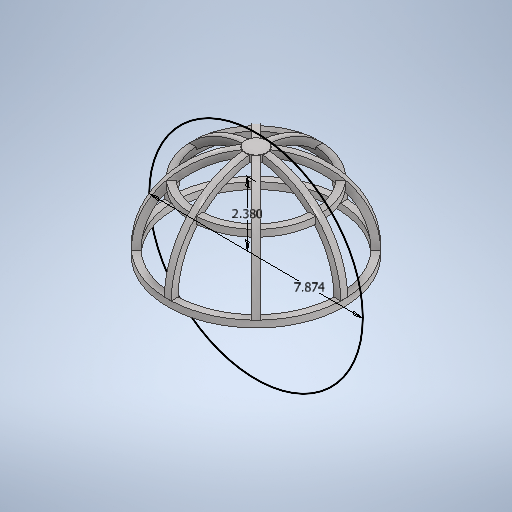
# Autodesk Inventor part: Dome
Saved by Autodesk Inventor 2025.1 (Build 291241000, 241)
## iProperties
Created: 2024-11-09
Part Number: Dome
Material: Steel, Mild, Welded
Document SubType Name: Modeling
Designer: monos
Density: 7.85 g/cm^3
Appearance: Weld - Steel Mild
Mass: 971.885 g
Surface Area: 500.62 cm^2
Volume: 123.807 cm^3
Author: monos
Autodesk Inventor part; units mm, degrees
sketch "200mm Measuring Ring" plane through (0, 0, 0) normal (0, 0, 1) x (1, 0, 0)
  circle A0 centre (0, 0) radius 100
  dimension "d4" = 200
  constraints: 1 centre point, 1 coincident
  measures "d4" diameter of A0
sketch "Sketch1" plane through (0, 0, 0) normal (0, 1, 0) x (-1, 0, 0)
  circle A0 centre (0, 0) radius 82.55
  circle A1 centre (0, 0) radius 76.2
  dimension "base_outer_d" = 165.1
  dimension "base_inner_d" = 152.4
  constraints: 2 centre point, 2 coincident
  measures "base_outer_d" diameter of A0
  measures "base_inner_d" diameter of A1
extrude "Extrusion1" add sketch "Sketch1" along normal blind 6.35
sketch "Sketch3" plane through (0, 0, 0) normal (1, 0, 0) x (0, 1, 0)
  line L0 (6.35, -82.55) -> (6.35, 82.55) projected
  arc A0 (88.9, 0) -> (6.35, 82.55) centre (6.35, 0) ccw
  line L1 (6.35, 0) -> (88.9, 0) construction
  line L2 (6.35, 0) -> (6.35, 82.55) construction
  arc A1 (82.55, 0) -> (6.35, 76.2) centre (6.35, 0) ccw
  arc A2 (6.35, -82.55) -> (88.9, 0) centre (6.35, 0) ccw
  arc A3 (6.35, -76.2) -> (82.55, 0) centre (6.35, 0) ccw
  line L3 (88.9, 0) -> (82.55, 0)
  line L4 (6.35, 82.55) -> (6.35, 76.2)
  line L5 (6.35, -82.55) -> (6.35, -76.2)
  line L6 (88.9, 0) -> (82.55, 0)
  point P0 (0, 0)
  point P1 (6.35, 76.2)
  dimension "d5" = 90
  dimension "d6" = 76.2
  dimension "d7" = 76.2
  constraints: 12 end point, 8 point on circle, 4 centre point, 4 collinear, 3 coincident, 3 point on line, 1 midpoint
  measures "d5" angle of L1 L2
  measures "d6" radius of A1
  measures "d7" radius of A3
extrude "Extrusion2" add sketch "Sketch3" along normal mid plane 6.35 contours L0 A3 L3 A2 | L3 A1 L0 A0
sketch "Sketch4" plane through (0, 0, 0) normal (0, 0, 1) x (1, 0, 0)
  line L0 (82.55, 6.35) -> (-82.55, 6.35) projected
  arc A0 (0, 88.9) -> (-82.55, 6.35) centre (0, 6.35) ccw
  arc A1 (0, 82.55) -> (-76.2, 6.35) centre (0, 6.35) ccw
  line L1 (-82.55, 6.35) -> (-76.2, 6.35)
  line L2 (0, 88.9) -> (0, 82.55)
  arc A2 (82.55, 6.35) -> (0, 88.9) centre (0, 6.35) ccw
  arc A3 (76.2, 6.35) -> (0, 82.55) centre (0, 6.35) ccw
  line L3 (0, 88.9) -> (0, 82.55)
  line L4 (76.2, 6.35) -> (82.55, 6.35)
  line L5 (82.55, 6.35) -> (76.2, 6.35)
  line L6 (-76.2, 6.35) -> (-82.55, 6.35)
  line L7 (0, 88.9) -> (0, 82.55)
  point P0 (0, 0)
  dimension "d8" = 76.2
  dimension "d9" = 76.2
  constraints: 14 end point, 8 point on circle, 4 centre point, 4 collinear, 3 coincident, 2 point on line, 1 horizontal, 1 midpoint, 1 perpendicular, 1 vertical
  measures "d8" radius of A1
  measures "d9" radius of A3
extrude "Extrusion3" add sketch "Sketch4" along normal mid plane 6.35 contours L0 A3 L2 A2 | L2 A1 L0 A0
ref_plane "Work Plane1" through (0, 0, 0) normal (-0.7071, 0, 0.7071) x (0, -1, 0)
sketch "Sketch5" plane through (0, 0, 0) normal (-0.7071, 0, 0.7071) x (0, -1, 0)
  line L0 (-6.35, -61.2311) -> (-6.35, 61.2311) projected
  line L1 (0, 82.55) -> (-6.35, 82.55) projected
  arc A0 (-6.35, 82.55) -> (-88.9, 0) centre (-6.35, 0) ccw
  line L2 (-6.35, 65.7212) -> (-6.35, 53.8815) projected
  arc A1 (-6.35, 76.2) -> (-82.55, 0) centre (-6.35, 0) ccw
  arc A2 (-88.9, 0) -> (-6.35, -82.55) centre (-6.35, 0) ccw
  arc A3 (-82.55, 0) -> (-6.35, -76.2) centre (-6.35, 0) ccw
  line L3 (-88.9, 0) -> (-82.55, 0)
  line L4 (-6.35, -82.55) -> (-6.35, -76.2)
  line L5 (-6.35, 76.2) -> (-6.35, 82.55)
  line L6 (0, 82.55) -> (0, -82.55) projected
  point P0 (0, 0)
  point P1 (-6.35, 89.825)
  point P2 (-6.35, -53.8815)
  point P3 (-82.55, 0)
  dimension "d14" = 76.2
  dimension "d15" = 76.2
  constraints: 8 point on circle, 6 end point, 4 centre point, 3 coincident, 3 point on line, 1 horizontal, 1 midpoint, 1 parallel, 1 perpendicular
  measures "d14" radius of A1
  measures "d15" radius of A3
extrude "Extrusion4" add sketch "Sketch5" along normal mid plane 6.35
ref_plane "Work Plane3" through (0, 0, 0) normal (0.7071, 0, 0.7071) x (0, 1, 0)
sketch "Sketch7" plane through (0, 0, 0) normal (0.7071, 0, 0.7071) x (0, 1, 0)
  line L0 (6.35, 0) -> (6.35, -53.8815) projected
  line L1 (6.35, -82.55) -> (6.35, -60.5735) projected
  arc A0 (6.35, -82.55) -> (88.9, 0) centre (6.35, 0) ccw
  arc A1 (6.35, -76.2) -> (82.55, 0) centre (6.35, 0) ccw
  line L2 (6.35, 60.5735) -> (6.35, 82.55) projected
  arc A2 (88.9, 0) -> (6.35, 82.55) centre (6.35, 0) ccw
  arc A3 (82.55, 0) -> (6.35, 76.2) centre (6.35, 0) ccw
  line L3 (88.9, 0) -> (82.55, 0)
  line L4 (6.35, -82.55) -> (6.35, -76.2)
  line L5 (6.35, 82.55) -> (6.35, 76.2)
  point P0 (82.55, 0)
  point P1 (6.35, -76.2)
  point P2 (6.35, 76.2)
  dimension "d27" = 76.2
  dimension "d28" = 76.2
  constraints: 8 point on circle, 6 end point, 4 centre point, 3 coincident, 2 collinear, 1 horizontal
  measures "d27" radius of A1
  measures "d28" radius of A3
extrude "Extrusion7" add sketch "Sketch7" along normal mid plane 6.35
ref_plane "Top Disk" through (0, 88.9, 0) normal (0, 1, 0) x (1, 0, 0)
sketch "Sketch8" plane through (0, 88.9, 0) normal (0, 1, 0) x (1, 0, 0)
  line L0 (3.175, -1.3151) -> (0, 0) projected
  circle A0 centre (0, 0) radius 10
  dimension "upper_example_d" = 20
  constraints: 1 centre point, 1 coincident
  measures "upper_example_d" diameter of A0
extrude "Extrusion8" add sketch "Sketch8" against normal blind 6.35
ref_plane "Work Plane5" through (0, 60.452, 0) normal (0, 1, 0) x (-1, 0, 0)
sketch "Sketch9" plane through (0, 60.452, 0) normal (0, 1, 0) x (-1, 0, 0)
  line L0 (0, 0) -> (-7.6651, 3.175) projected
  circle A0 centre (0, 0) radius 59.4462
  line L1 (3.175, -7.6651) -> (0, 0) projected
  circle A1 centre (0, 0) radius 53.0962
  dimension "middle_outer_d" = 118.8923
  dimension "middle_inner_d" = 106.1924
  constraints: 2 centre point, 1 coincident
  measures "middle_outer_d" diameter of A0
  measures "middle_inner_d" diameter of A1
extrude "Middle ring" add sketch "Sketch9" along normal mid plane 6.35
sketch "Sketch10" plane through (0, 0, 0) normal (0, 0, 1) x (1, 0, 0)
  line L0 (0, 0) -> (0, 60.452)
  dimension "height" = 60.452
  constraints: 2 end point, 1 vertical
  measures "height" distance of L0.start L0.end
sketch "Sketch13" plane through (0, 78.74, 0) normal (0, 1, 0) x (-1, 0, 0)
  line L0 (0, 0) -> (-7.6651, 3.175)
  circle A0 centre (0, 0) radius 33.233
  line L1 (3.175, -7.6651) -> (0, 0)
  circle A1 centre (0, 0) radius 26.883
  dimension "d49" = 66.466
  dimension "d48" = 53.766
  constraints: 4 end point, 2 centre point, 1 coincident
  measures "d49" diameter of A0
  measures "d48" diameter of A1
sketch "Sketch11" plane through (0, 72.39, 0) normal (0, 1, 0) x (-1, 0, 0)
  line L0 (7.6651, 3.175) -> (0, 0) projected
  circle A0 centre (0, 0) radius 38.1
  dimension "d41" = 76.2
  constraints: 1 centre point, 1 coincident
  measures "d41" diameter of A0
body "Solid1"
